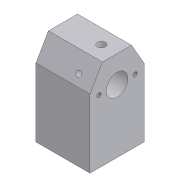
# Autodesk Inventor part: 23-0064 Diode holder
Saved by Autodesk Inventor 2022.4 (Build 264492000, 492)
## iProperties
Category: -
Company: Universiteit van Amsterdam
Created: 2023-08-21
Part Number: 23-0064 Diode holder
Material: Stainless Steel 316 (X5CrNiMo17.12.2)
Document SubType Name: Modeling
Designer: RbSrWorkstation1
Density: 8 g/cm^3
Appearance: Steel
User Status: Work in Progress
Author: RbSrWorkstation1
Revision Number: A
Autodesk Inventor part; units mm, degrees
ref_plane "XZ Plane" through (0, 0, 0) normal (0, 1, 0) x (-1, 0, 0)
ref_plane "XY Plane" through (0, 0, 0) normal (0, 0, 1) x (1, 0, 0)
sketch "Sketch1" plane through (0, 0, 0) normal (0, 1, 0) x (-1, 0, 0)
  line L0 (-15, -15) -> (15, -15)
  line L1 (15, -15) -> (15, 15)
  line L2 (15, 15) -> (-15, 15)
  line L3 (-15, 15) -> (-15, -15)
  line L4 (-15, -15) -> (15, 15) construction
  line L5 (15, -15) -> (-15, 15) construction
  point P0 (0, 0)
  dimension "d0" = 30
  dimension "d1" = 30
  constraints: 12 end point, 2 midpoint, 2 parallel, 1 horizontal, 1 perpendicular
  measures "d0" distance of L0.end L1.end
  measures "d1" distance of L1.end L2.end
extrude "Extrusion1" add sketch "Sketch1" along normal blind 50
sketch "Sketch2" plane through (15, 0, 15) normal (1, 0, 0) x (0, 0, -1)
  line L0 (15, 0) -> (15, 35) construction
  line L1 (0, 0) -> (30, 0) projected
  circle A0 centre (15, 35) radius 6
  dimension "d4" = 35
  dimension "d6" = 12
  constraints: 2 end point, 1 centre point, 1 coincident, 1 vertical
  measures "d4" distance of L0.start L0.end
  measures "d6" diameter of A0
extrude "Extrusion2" cut sketch "Sketch2" against normal through all
sketch "Sketch7" plane through (0, 50, 0) normal (0, 1, 0) x (1, 0, 0)
  line L0 (15, -15) -> (15, 15) projected
  line L1 (6.5, 0) -> (6.35, 0)
  circle A0 centre (6.35, 0) radius 2.25
  point P0 (0, 0)
  dimension "d33" = 4.5
  dimension "d119" = 8.65
  constraints: 2 end point, 1 centre point, 1 coincident
  measures "d33" diameter of A0
  measures "d119" distance from line of L1.end L0
extrude "Extrusion7" cut sketch "Sketch7" against normal blind 12
ref_plane "Work Plane1" through (6.35, 0, 0) normal (1, 0, 0) x (0, 1, 0)
sketch "Sketch14" plane through (6.35, 0, 0) normal (1, 0, 0) x (0, 1, 0)
  line L0 (50, -15) -> (50, 15) projected
  circle A0 centre (35, 0) radius 6 projected
  line L1 (50, 0) -> (35, 0)
  line L2 (35, 0) -> (52.3205, -30)
  line L3 (35, 0) -> (61.673, 0)
  line L4 (35, 0) -> (36.7321, 0)
  line L5 (36.7321, 0) -> (54.0526, -30)
  line L6 (54.0526, -30) -> (52.3205, -30)
  line L7 (52, -6.9171) -> (34.5359, -17)
  line L8 (34.5359, -17) -> (52, -17)
  line L9 (52, -17) -> (52, -6.9171)
  line L10 (0, -15) -> (50, -15) projected
  line L11 (0, -15) -> (50, -15) projected
  point P0 (0, 0)
  point P1 (36.7321, 0)
  point P2 (38, -15)
  dimension "d55" = 60
  dimension "d57" = 120
  dimension "d72" = 1.5
  dimension "d73" = 30
  dimension "d112" = 2
  dimension "d113" = 2
  dimension "d114" = 12
  constraints: 18 end point, 3 horizontal, 3 point on line, 2 perpendicular, 1 midpoint, 1 parallel
  measures "d55" angle of L1 L2
  measures "d57" angle of L4 L5
  measures "d72" distance from line of L5.end L2
  measures "d73" vertical distance of L4.end L5.end
  measures "d112" distance between parallel lines of L9 L0
  measures "d113" distance between parallel lines of L8 L10
  measures "d114" distance from line of point (38, -15) L0
revolve "Revolution1" cut sketch "Sketch14" angle 360 about axis through (6.35, 35, 0) along (0, 0.5, -0.8660254) contours L10 L2 L7 L5 | L5 L8 L2 L10 | L7 L2 A0 L5 | L5 L6 L2 L8 | A0 L2 L1 L5
extrude "Extrusion11" cut sketch "Sketch14" along normal blind 99 and the other way blind 99 contours L10 L5 L7 L0 | L0 L7 L9 L8 L5 L10 | L10 L2 L7 L5 | L5 L8 L2 L10 | L10 L7 L2 | L2 L8 L7 L10
mirror "Mirror4" about plane through (0, 0, 0) normal (0, 0, 1) of "Revolution1", "Extrusion11"
sketch "Sketch19" plane through (0, 0, 0) normal (0, -1, 0) x (1, 0, 0)
  point P0 (0, 0)
  point P1 (-10, 10)
  point P2 (10, -10)
  dimension "d97" = 10
  dimension "d98" = 10
  dimension "d99" = 10
  dimension "d100" = 10
  measures "d97" horizontal distance of point (-10, 10) point (0, 0)
  measures "d98" horizontal distance of point (-10, 10) point (0, 0)
  measures "d99" horizontal distance of point (10, -10) point (0, 0)
  measures "d100" horizontal distance of point (0, 0) point (10, -10)
hole "Hole2" at (-10, 0, 10) at (10, 0, -10) direction (0, 1, 0) diameter 4.134 depth 15 tip angle 118 thread size "M5x0.8" class "6H" standard "ISO Metric profile"
sketch "Sketch20" plane through (0, 0, 0) normal (0, -1, 0) x (1, 0, 0)
  point P0 (0, 0)
  point P1 (10, 10)
  point P2 (-10, -10)
  dimension "d108" = 10
  dimension "d109" = 10
  dimension "d110" = 10
  dimension "d111" = 10
  measures "d108" horizontal distance of point (10, 10) point (0, 0)
  measures "d109" horizontal distance of point (10, 10) point (0, 0)
  measures "d110" horizontal distance of point (0, 0) point (-10, -10)
  measures "d111" horizontal distance of point (0, 0) point (-10, -10)
hole "Hole3" at (10, 0, 10) at (-10, 0, -10) direction (0, 1, 0) diameter 4 depth 15 tip angle 118
sketch "Sketch21" plane through (15, 0, 15) normal (1, 0, 0) x (0, 0, -1)
  line L0 (0, 0) -> (30, 0) projected
  circle A0 centre (15, 35) radius 6 projected
  point P0 (15, 0)
  point P1 (5, 35)
  point P2 (25, 35)
  point P3 (15, 0)
  point P4 (15, 0)
  dimension "d127" = 10
  dimension "d128" = 10
  constraints: 2 horizontal alignment, 2 midpoint
  measures "d127" horizontal distance of point (15, 0) point (5, 35)
  measures "d128" horizontal distance of point (15, 0) point (25, 35)
hole "Hole4" at (15, 35, 10) at (15, 35, -10) direction (-1, 0, 0) diameter 2.459 depth 9 tip angle 118 thread size "M3x0.5" class "6H" standard "ISO Metric profile"
equation "\"d99\" = d98"
equation "\"d100\" = d97"
equation "\"d110\" = d109"
equation "\"d111\" = d108"
body "Solid1"
